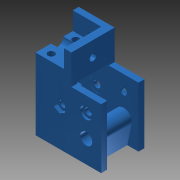
# Autodesk Inventor part: YIdlerBlockLeft
Saved by Autodesk Inventor 2015 SP1 (Build 190203100, 203)
## iProperties
Category: Print
Created: 2014-08-14
Part Number: YIdlerBlockLeft
Material: ABS Plastic
Document SubType Name: Modeling
Designer: t_clevj
Density: 1.06 g/cm^3
Appearance: Cyan
Mass: 26.9786 g
Surface Area: 144.798 cm^2
Volume: 25.4515 cm^3
Vendor: Jack
Author: Jack; Zelogik
Title: Y Idler Block Left
Autodesk Inventor part; units mm, degrees
ref_plane "YZ Plane" through (0, 0, 0) normal (1, 0, 0) x (0, 1, 0)
ref_plane "XZ Plane" through (0, 0, 0) normal (0, 1, 0) x (-1, 0, 0)
ref_plane "XY Plane" through (0, 0, 0) normal (0, 0, 1) x (1, 0, 0)
sketch "Sketch1" plane through (0, 0, 0) normal (0, 1, 0) x (-1, 0, 0)
  line L0 (0, 0) -> (44, 0)
  line L1 (44, 0) -> (44, 60)
  line L2 (44, 60) -> (20, 60)
  line L3 (20, 60) -> (20, 40)
  line L4 (20, 40) -> (0, 40)
  line L5 (0, 40) -> (0, 0)
  dimension "d0" = 44
  dimension "d1" = 60
  dimension "d2" = 24
  dimension "d3" = 20
  constraints: 12 end point, 4 perpendicular, 2 horizontal
  measures "d0" distance of L0.start L0.end
  measures "d1" distance of L0.end L1.end
  measures "d2" distance of L1.end L2.end
  measures "d3" distance of L2.end L3.end
extrude "BaseBottom" add sketch "Sketch1" along normal blind 4
sketch "Sketch2" plane through (0, 4, 0) normal (0, 1, 0) x (1, 0, 0)
  line L0 (0, 0) -> (-44, 0) projected
  line L1 (-44, 0) -> (-44, -60) projected
  line L2 (-44, -60) -> (-20, -60) projected
  line L3 (-20, -60) -> (-20, -40) projected
  line L4 (-20, -40) -> (0, -40) projected
  line L5 (0, -40) -> (0, 0) projected
  circle A0 centre (-10, -15) radius 5.5
  line L6 (-4.6151, -13.8808) -> (-7.5, 0)
  line L7 (-15.3849, -13.8808) -> (-12.5, 0)
  line L8 (-20, -41) -> (-44, -41)
  arc A1 (-34, -15.7805) -> (-37.798, -20) centre (-28, -25) ccw
  line L9 (-34, 0) -> (-34, -15.7805)
  line L10 (-37.798, -20) -> (-44, -20)
  dimension "d6" = 11
  dimension "d7" = 10
  dimension "d8" = 15
  dimension "d9" = 5
  dimension "d10" = 7.5
  dimension "d11" = 1
  dimension "d12" = 22
  dimension "d13" = 25
  dimension "d14" = 16
  dimension "d15" = 10
  dimension "d16" = 20
  constraints: 10 end point, 6 point on line, 4 point on circle, 2 centre point, 2 perpendicular, 2 tangent, 1 vertical
  measures "d6" diameter of A0
  measures "d7" distance from line of L5 A0.centre
  measures "d8" distance from line of L0 A0.centre
  measures "d9" distance of L6.end L7.end
  measures "d10" distance from line of L5 L6.end
  measures "d11" distance between parallel lines of L4 L8
  measures "d12" diameter of A1
  measures "d13" distance from line of L0 A1.centre
  measures "d14" distance from line of L1 A1.centre
  measures "d15" distance between parallel lines of L1 L9
  measures "d16" distance between parallel lines of L0 L10
extrude "SpannerMaterial" add sketch "Sketch2" along normal blind 21 contours L6 A0 L7 L0 | A0 | L9 A1 L10 L1 L0 | L3 L2 L1 L8
sketch "Sketch3" plane through (0, 25, 0) normal (0, 1, 0) x (1, 0, 0)
  line L0 (-34, 0) -> (-44, 0) projected
  line L1 (-34, 0) -> (0, 0)
  line L2 (0, 0) -> (0, -40)
  line L3 (0, -40) -> (-20, -40)
  line L4 (-20, -40) -> (-20, -60)
  line L5 (-20, -60) -> (-44, -60)
  line L6 (-44, -60) -> (-44, 0)
  constraints: 12 end point, 5 perpendicular, 1 horizontal
extrude "TopSurface" add sketch "Sketch3" along normal blind 4
sketch "Sketch4" plane through (-44, 0, 0) normal (-1, 0, 0) x (0, 0, 1)
  line L0 (0, 0) -> (60, 0) projected
  line L1 (60, 0) -> (60, 29) projected
  line L2 (60, 25) -> (48, 25)
  line L3 (48, 25) -> (48, 0)
  dimension "d21" = 12
  dimension "d22" = 25
  constraints: 4 end point, 2 point on line, 1 horizontal, 1 perpendicular
  measures "d21" distance of L2.start L2.end
  measures "d22" distance of L2.end L3.end
extrude "YRodNotch" cut sketch "Sketch4" against normal blind 19
sketch "Sketch6" plane through (-44, 0, 0) normal (-1, 0, 0) x (0, 0, 1)
  line L0 (48, 25) -> (60, 25) projected
  line L1 (48, 0) -> (48, 25) projected
  circle A0 centre (48, 14.5) radius 4.1
  dimension "d29" = 8.2
  dimension "d30" = 10.5
  constraints: 1 centre point, 1 point on line
  measures "d29" diameter of A0
  measures "d30" distance from line of L0 A0.centre
extrude "YRodHole" cut sketch "Sketch6" against normal up to surface (19 mm away)
ref_plane "Work Plane1" through (-44, 29, 50) normal (0, 0, 1) x (1, 0, 0)
sketch "Sketch21" plane through (0, 0, 0) normal (0, -1, 0) x (1, 0, 0)
  arc A0 (-4.6151, 13.8808) -> (-15.3849, 13.8808) centre (-10, 15) ccw projected
  arc A1 (-4.6151, 13.8808) -> (-15.3849, 13.8808) centre (-10, 15) ccw projected
hole "FrameBoltBackTop" at (-10, 0, 15) direction (0, 1, 0) diameter 4.5 end up to face face through (-21.3333, 29, 13.3333) facing (0, 1, 0) counterbore diameter 8 counterbore depth 25
sketch "Sketch22" plane through (0, 29, 0) normal (0, 1, 0) x (1, 0, 0)
  line L0 (-44, 0) -> (-44, -60) projected
  line L1 (0, 0) -> (-44, 0) projected
  point P0 (-28, -25)
  dimension "d94" = 25
  dimension "d95" = 16
  measures "d94" distance from line of L1 point (-28, -25)
  measures "d95" distance from line of L0 point (-28, -25)
hole "BearingHoleInner" at (-28, 29, 25) direction (0, -1, 0) diameter 4.5 end up to face face through (-36, 0, 29.3333) facing (0, -1, 0) counterbore diameter 8 counterbore depth 1.5
sketch "Sketch23" plane through (0, 0, 0) normal (0, -1, 0) x (1, 0, 0)
  line L0 (0, 0) -> (-44, 0) projected
  line L1 (0, 40) -> (0, 0) projected
  point P0 (-10, 30)
  dimension "d103" = 30
  dimension "d104" = 10
  measures "d103" distance from line of L0 point (-10, 30)
  measures "d104" distance from line of L1 point (-10, 30)
hole "BearingHoleOuter" at (-10, 0, 30) direction (0, 1, 0) diameter 4.5 end up to face face through (-40, 29, 28.3333) facing (0, 1, 0) counterbore diameter 8 counterbore depth 1.5
sketch "Sketch24" plane through (0, 29, 0) normal (0, 1, 0) x (1, 0, 0)
  circle A0 centre (-10, -30) radius 2.25 projected
  line L0 (-10, -34.2724) -> (-13.7, -32.1362)
  line L1 (-13.7, -32.1362) -> (-13.7, -27.8638)
  line L2 (-13.7, -27.8638) -> (-10, -25.7276)
  line L3 (-10, -25.7276) -> (-6.3, -27.8638)
  line L4 (-6.3, -27.8638) -> (-6.3, -32.1362)
  line L5 (-6.3, -32.1362) -> (-10, -34.2724)
  dimension "d112" = 7.4
  constraints: 12 end point, 1 coincident, 1 vertical, 13 other
  measures "d112" distance between parallel lines of L1 L4
extrude "BearingHoleOuterNutTrap" cut sketch "Sketch24" against normal blind 3.2
sketch "Sketch25" plane through (0, 0, 0) normal (0, -1, 0) x (1, 0, 0)
  circle A0 centre (-28, 25) radius 2.25 projected
  line L0 (-28, 29.2724) -> (-24.3, 27.1362)
  line L1 (-24.3, 27.1362) -> (-24.3, 22.8638)
  line L2 (-24.3, 22.8638) -> (-28, 20.7276)
  line L3 (-28, 20.7276) -> (-31.7, 22.8638)
  line L4 (-31.7, 22.8638) -> (-31.7, 27.1362)
  line L5 (-31.7, 27.1362) -> (-28, 29.2724)
  dimension "d115" = 7.4
  constraints: 12 end point, 1 coincident, 1 vertical, 13 other
  measures "d115" distance between parallel lines of L1 L4
extrude "BearingHoleInnerNutTrap" cut sketch "Sketch25" against normal blind 2.5
sketch "Sketch28" plane through (-25, 0, 0) normal (-1, 0, 0) x (0, 0, 1)
  line L0 (60, 25) -> (60, 0) projected
  arc A0 (48, 18.6) -> (48, 10.4) centre (48, 14.5) ccw projected
  circle A1 centre (50, 14.5) radius 2.25
  point P0 (0, 0)
  dimension "d125" = 4.5
  dimension "d126" = 10
  constraints: 1 centre point, 1 horizontal alignment
  measures "d125" diameter of A1
  measures "d126" distance from line of L0 A1.centre
extrude "Extrusion22" cut sketch "Sketch28" against normal up to next
sketch "Sketch29" plane through (-44, 0, 48) normal (0, 0, 1) x (1, 0, 0)
  line L0 (19, 0) -> (0, 0) projected
  line L1 (0, 18.6) -> (19, 18.6) projected
  line L2 (19, 18.6) -> (19, 25) projected
  line L3 (0, 25) -> (19, 25) projected
  line L4 (0, 18.6) -> (0, 25) projected
  circle A0 centre (6, 21) radius 2.25
  circle A1 centre (6, 4.5) radius 2.25
  line L5 (0, 0) -> (0, 10.4) projected
  point P0 (44, 0)
  dimension "d129" = 4.5
  dimension "d131" = 4.5
  dimension "d132" = 4
  dimension "d167" = 6
  constraints: 2 centre point, 1 equal radius, 1 vertical alignment
  measures "d129" diameter of A0
  measures "d131" distance from line of L0 A1.centre
  measures "d132" distance from line of L3 A0.centre
  measures "d167" distance from line of L5 A1.centre
extrude "Extrusion23" cut sketch "Sketch29" against normal up to surface (7 mm away) contours A0 | A1
sketch "Sketch30" plane through (-20, 25, 41) normal (0, 0, -1) x (-1, 0, 0)
  arc A0 (20.1937, -21) -> (15.8063, -21) centre (18, -20.5) ccw projected
  circle A1 centre (18, -4) radius 2.25 projected
  line L0 (22.2724, -4) -> (20.1362, -7.7)
  line L1 (20.1362, -7.7) -> (15.8638, -7.7)
  line L2 (15.8638, -7.7) -> (13.7276, -4)
  line L3 (13.7276, -4) -> (15.8638, -0.3)
  line L4 (15.8638, -0.3) -> (20.1362, -0.3)
  line L5 (20.1362, -0.3) -> (22.2724, -4)
  line L6 (22.2724, -20.5) -> (20.1362, -24.2)
  line L7 (20.1362, -24.2) -> (15.8638, -24.2)
  line L8 (15.8638, -24.2) -> (13.7276, -20.5)
  line L9 (13.7276, -20.5) -> (15.8638, -16.8)
  line L10 (15.8638, -16.8) -> (20.1362, -16.8)
  line L11 (20.1362, -16.8) -> (22.2724, -20.5)
  point P0 (-20, -25)
  dimension "d136" = 7.4
  constraints: 24 end point, 2 coincident, 2 horizontal, 1 parallel, 26 other
  measures "d136" distance between parallel lines of L7 L10
extrude "Extrusion24" cut sketch "Sketch30" against normal blind 4 and the other way blind 4
ref_plane "Work Plane2" through (-44, 29, 50) normal (0, 0, 1) x (1, 0, 0)
sketch "Sketch31" plane through (-44, 29, 50) normal (0, 0, 1) x (1, 0, 0)
  line L0 (24, -12.25) -> (24, -16.75) projected
  line L1 (19, -16.75) -> (19, -12.25) projected
  line L2 (19, -10.4) -> (19, -18.6) projected
  line L3 (19, -14.5) -> (19, -10.25)
  line L4 (19, -10.4) -> (19, -4) projected
  line L5 (19, -14.5) -> (19, -18.75)
  line L6 (19, -29) -> (19, -18.6) projected
  line L7 (19, -18.75) -> (21.5, -16.75)
  line L8 (21.5, -16.75) -> (21.5, -12.25)
  line L9 (21.5, -12.25) -> (19, -10.25)
  line L10 (19, -14.5) -> (21.5, -14.5)
  point P0 (44, -29)
  dimension "d142" = 4.25
  dimension "d143" = 4.25
  dimension "d144" = 2.5
  dimension "d145" = 4.5
  constraints: 12 end point, 2 midpoint, 2 point on line, 1 equal length, 1 parallel
  measures "d142" distance of L3.start L3.end
  measures "d143" distance of L3.start L5.end
  measures "d144" distance between parallel lines of L3 L8
  measures "d145" distance of L7.end L8.end
revolve "Revolution4" cut sketch "Sketch31" angle 360 about axis through (-25, 14.5, 50) along (1, 0, 0) contours L1 L10 L8 L7 L5 L2
sketch "Sketch33" plane through (-44, 25, 48) normal (0, -1, 0) x (1, 0, 0)
  line L0 (19, 0) -> (19, 12) projected
  line L1 (0, 12) -> (19, 12) projected
  circle A0 centre (13.9, 2) radius 2.25
  line L2 (24, 12) -> (24, -8) projected
  point P0 (44, -48)
  dimension "d149" = 4.5
  dimension "d151" = 5.1
  dimension "d152" = 10
  constraints: 1 centre point
  measures "d149" diameter of A0
  measures "d151" distance from line of L0 A0.centre
  measures "d152" distance from line of L1 A0.centre
extrude "Extrusion26" cut sketch "Sketch33" against normal up to surface (4 mm away)
ref_plane "Work Plane3" through (-30.1, 0, 0) normal (-1, 0, 0) x (0, 0, 1)
sketch "Sketch34" plane through (-30.1, 0, 0) normal (-1, 0, 0) x (0, 0, 1)
  line L0 (52.25, 25) -> (48, 25) projected
  line L1 (50.125, 25) -> (54.375, 25)
  line L2 (48, 25) -> (60, 25) projected
  line L3 (54.375, 25) -> (52.25, 27.5)
  line L4 (52.25, 25) -> (52.25, 29) projected
  line L5 (52.25, 27.5) -> (50.125, 27.5)
  line L6 (50.125, 27.5) -> (50.125, 25)
  point P0 (0, 0)
  dimension "d156" = 4.25
  dimension "d157" = 2.5
  constraints: 8 end point, 2 point on line, 1 horizontal, 1 midpoint, 1 perpendicular
  measures "d156" distance of L1.start L1.end
  measures "d157" distance from line of L1 L3.end
revolve "Revolution5" cut sketch "Sketch34" angle 360 about axis through (-30.1, 27.5, 50.125) along (0, -1, 0)
sketch "Sketch35" plane through (-44, 25, 48) normal (0, -1, 0) x (1, 0, 0)
  arc A0 (17.5806, 0) -> (10.2194, 0) centre (13.9, 2.125) ccw projected
  arc A1 (10.2194, 0) -> (17.5806, 0) centre (13.9, 2.125) ccw projected
  point P0 (44, -48)
  constraints: 1 other
extrude "Extrusion27" cut sketch "Sketch35" along normal blind 6
sketch "Sketch36" plane through (0, 4, 0) normal (0, 1, 0) x (1, 0, 0)
  circle A0 centre (-10, -30) radius 4 projected
  circle A1 centre (-10, -30) radius 4.75
  dimension "d161" = 9.5
  constraints: 1 centre point, 1 coincident
  measures "d161" diameter of A1
extrude "Extrusion28" cut sketch "Sketch36" against normal blind 0.25 contours A0 | A1
sketch "Sketch37" plane through (0, 25, 0) normal (0, -1, 0) x (1, 0, 0)
  circle A0 centre (-28, 25) radius 2.25 projected
  arc A1 (-37.798, 20) -> (-34, 15.7805) centre (-28, 25) ccw projected
  circle A2 centre (-28, 25) radius 4.75
  dimension "d164" = 9.5
  constraints: 1 centre point, 1 coincident
  measures "d164" diameter of A2
extrude "Extrusion29" cut sketch "Sketch37" against normal blind 0.25
body "Solid1"
